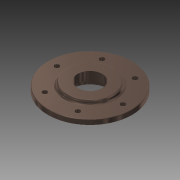
# Autodesk Inventor part: 主动轴大端盖
Saved by Autodesk Inventor 2015 (Build 190159000, 159)
## iProperties
Created: 2017-05-09
Part Number: 主动轴大端盖
Material: 常规
Document SubType Name: Modeling
Designer: Administrator
Density: 1 g/cm^3
Appearance: 铁灰色 - 仿古抛光
Author: Administrator
Autodesk Inventor part; units mm, degrees
ref_plane "YZ Plane" through (0, 0, 0) normal (1, 0, 0) x (0, 1, 0)
ref_plane "XZ Plane" through (0, 0, 0) normal (0, 1, 0) x (-1, 0, 0)
ref_plane "XY Plane" through (0, 0, 0) normal (0, 0, 1) x (1, 0, 0)
sketch "草图1" plane through (0, 0, 0) normal (0, 0, 1) x (1, 0, 0)
  circle A0 centre (0, 0) radius 70
  dimension "d0" = 140
  constraints: 1 centre point, 1 coincident
  measures "d0" diameter of A0
extrude "拉伸1" add sketch "草图1" along normal blind 8
sketch "草图2" plane through (0, 0, 0) normal (0, 0, -1) x (-1, 0, 0)
  circle A0 centre (0, 0) radius 40
  circle A1 centre (0, 0) radius 30
  dimension "d3" = 80
  dimension "d4" = 60
  constraints: 2 centre point, 2 coincident
  measures "d3" diameter of A0
  measures "d4" diameter of A1
extrude "拉伸2" add sketch "草图2" along normal blind 12
sketch "草图3" plane through (0, 0, -12) normal (0, 0, -1) x (-1, 0, 0)
  circle A0 centre (0, 0) radius 40
  circle A1 centre (0, 0) radius 39
  dimension "d7" = 80
  dimension "d8" = 78
  constraints: 2 centre point, 2 coincident
  measures "d7" diameter of A0
  measures "d8" diameter of A1
extrude "拉伸3" cut sketch "草图3" against normal blind 4
fillet "圆角2" radius 1 1 edges at (-70, 0, 8)
sketch "草图5" plane through (0, 0, 8) normal (0, 0, 1) x (1, 0, 0)
  circle A0 centre (-55, 0) radius 4
  line L0 (0, 0) -> (-8.161, 0)
  dimension "d16" = 8
  dimension "d17" = 8.161
  dimension "d18" = 55
  constraints: 2 end point, 1 centre point, 1 horizontal, 1 point on line
  measures "d16" diameter of A0
  measures "d17" distance of L0.start L0.end
  measures "d18" distance of L0.start A0.centre
extrude "拉伸5" cut sketch "草图5" against normal through all
pattern_circular "环形阵列1" count 6 over 360 about axis through (0, 0, -10) along (0, 0, 1) of "拉伸5"
sketch "草图6" plane through (0, 0, 8) normal (0, 0, 1) x (1, 0, 0)
  circle A0 centre (0, 0) radius 40
  dimension "d24" = 80
  constraints: 1 centre point, 1 coincident
  measures "d24" diameter of A0
extrude "拉伸6" add sketch "草图6" along normal blind 6
sketch "草图7" plane through (0, 0, 14) normal (0, 0, 1) x (1, 0, 0)
  circle A0 centre (0, 0) radius 20.5
  dimension "d27" = 41
  constraints: 1 centre point, 1 coincident
  measures "d27" diameter of A0
extrude "拉伸7" cut sketch "草图7" against normal through all
fillet "圆角3" radius 3 2 edges at (-40, 0, 14) (-40, 0, 8)
